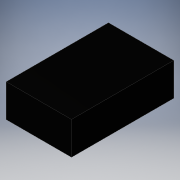
# Autodesk Inventor part: ESS REM10-0505S A
Saved by Autodesk Inventor 2016 SP2 (Build 200236200, 236)
## iProperties
Created: 2017-02-02
Part Number: ESS REM10-0505S A
Material: Generic
Document SubType Name: Modeling
Designer: eschr_000
Mass: 14 g
Surface Area: 23.5392 cm^2
Volume: 6.58451 cm^3
Density: 2.1262 g/cm^3
Appearance: Default
Author: eschr_000
Autodesk Inventor part; units mm, degrees
ref_plane "YZ Plane" through (0, 0, 0) normal (1, 0, 0) x (0, 1, 0)
ref_plane "XZ Plane" through (0, 0, 0) normal (0, 1, 0) x (-1, 0, 0)
ref_plane "XY Plane" through (0, 0, 0) normal (0, 0, 1) x (1, 0, 0)
sketch "Sketch2" plane through (0, 0, 0) normal (0, 1, 0) x (-1, 0, 0)
  line L0 (-10.15, 15.9) -> (10.15, 15.9)
  line L1 (10.15, 15.9) -> (10.15, -15.9)
  line L2 (10.15, -15.9) -> (-10.15, -15.9)
  line L3 (-10.15, -15.9) -> (-10.15, 15.9)
  line L4 (-10.15, 15.9) -> (10.15, -15.9) construction
  line L5 (10.15, 15.9) -> (-10.15, -15.9) construction
  point P0 (0, 0)
  dimension "d0" = 20.3
  dimension "d1" = 31.8
  constraints: 12 end point, 2 midpoint, 2 parallel, 1 horizontal, 1 perpendicular
  measures "d0" distance of L1.end L2.end
  measures "d1" distance of L2.end L0.start
extrude "Extrusion1" add sketch "Sketch2" along normal blind 10.2
body "Solid1"
